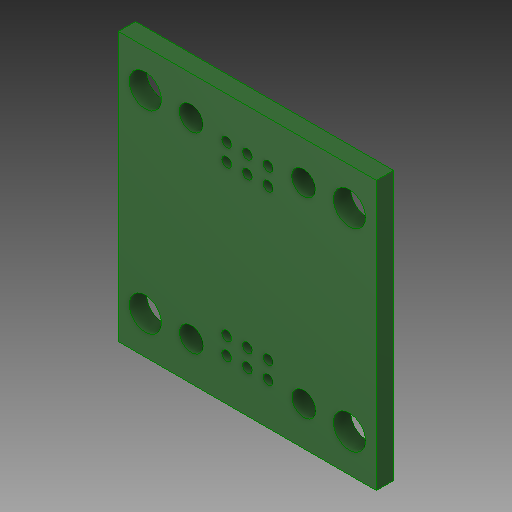
# Autodesk Inventor part: untitled.brd_Outline
Saved by Autodesk Inventor 2017 (Build 210142000, 142)
## iProperties
Created: 2022-08-30
Part Number: untitled.brd_Outline
Material: Generic
Document SubType Name: Modeling
Designer: Collin
Density: 1 g/cm^3
Appearance: Board Outline
Author: Collin
Autodesk Inventor part; units mm, degrees
ref_plane "YZ Plane" through (0, 0, 0) normal (1, 0, 0) x (0, 1, 0)
ref_plane "XZ Plane" through (0, 0, 0) normal (0, 1, 0) x (-1, 0, 0)
ref_plane "XY Plane" through (0, 0, 0) normal (0, 0, 1) x (1, 0, 0)
sketch "Sketch1" plane through (0, 0, 0) normal (0, 0, 1) x (1, 0, 0)
  line L0 (0, -0.5) -> (24, -0.5)
  line L1 (24, -0.5) -> (24, 24.5)
  line L2 (24, 24.5) -> (0, 24.5)
  line L3 (0, 24.5) -> (0, -0.5)
  circle A0 centre (13.93, 20.61) radius 0.45
  circle A1 centre (17.22, 20.91) radius 1.1
  circle A2 centre (6.75, 20.91) radius 1.1
  circle A3 centre (13.93, 19) radius 0.45
  circle A4 centre (12, 20.61) radius 0.45
  circle A5 centre (12, 19) radius 0.45
  circle A6 centre (10.07, 20.61) radius 0.45
  circle A7 centre (10.07, 19) radius 0.45
  circle A8 centre (10.07, 3.39) radius 0.45
  circle A9 centre (6.78, 3.1) radius 1.1
  circle A10 centre (17.25, 3.1) radius 1.1
  circle A11 centre (10.07, 5) radius 0.45
  circle A12 centre (12, 3.39) radius 0.45
  circle A13 centre (12, 5) radius 0.45
  circle A14 centre (13.93, 3.39) radius 0.45
  circle A15 centre (13.93, 5) radius 0.45
  circle A16 centre (2.5, 21) radius 1.5
  circle A17 centre (21.5, 21) radius 1.5
  circle A18 centre (21.5, 3) radius 1.5
  circle A19 centre (2.5, 3) radius 1.5
  constraints: 20 centre point, 8 end point
extrude "untitled.brd_Outline" add sketch "Sketch1" along normal blind 1.6
body "Solid1"
